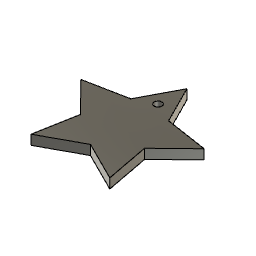
keychain v1 (Autodesk Fusion 360 design; units mm, degrees)
Autodesk Fusion 360 part; units mm, degrees
sketch "Sketch4" plane through (0, 0, 0) normal (0, 0, 1) x (1, 0, 0)
  line L0 (-14, 13) -> (26, 13)
  line L1 (26, 13) -> (26, -27)
  line L2 (26, -27) -> (-14, -27)
  line L3 (-14, -27) -> (-14, 13)
  line L4 (6, 11) -> (11.7842, -0.4932)
  line L5 (11.7842, -0.4932) -> (24.8229, -2.4867)
  line L6 (24.8229, -2.4867) -> (15.448, -11.6461)
  line L7 (15.448, -11.6461) -> (18, -25)
  line L8 (18, -25) -> (6, -19)
  line L9 (6, -19) -> (-5.9959, -25.493)
  line L10 (-5.9959, -25.493) -> (-3.6252, -12.5082)
  line L11 (-3.6252, -12.5082) -> (-13, -3)
  line L12 (-13, -3) -> (0.0021, -0.4393)
  line L13 (0.0021, -0.4393) -> (6, 11)
  constraint horizontal L0
  constraint vertical L1
  constraint horizontal L2
  constraint vertical L3
extrude "Extrude1" add sketch "Sketch4" along normal blind 3 contours L4 L5 L6 L7 L8 L9 L10 L11 L12 L13
cylinder "CylinderPrimitive1" cut diameter 2.33 height -3 placed x (1, 0, 0) y (0, 1, 0) z (0, 0, 1) at (5.6258, 2.3767, 3)
sketch "Sketch2" plane through (0, 0, 0) normal (0, 0, 1) x (1, 0, 0)
  line L0 (-22.5492, 19.9652) -> (17.4508, 19.9652)
  line L1 (17.4508, 19.9652) -> (17.4508, -20.0348)
  line L2 (17.4508, -20.0348) -> (-22.5492, -20.0348)
  line L3 (-22.5492, -20.0348) -> (-22.5492, 19.9652)
  constraint horizontal L0
  constraint vertical L1
  constraint horizontal L2
  constraint vertical L3
named bodies: "star2"
